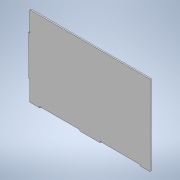
# Autodesk Inventor part: Base lateral
Saved by Autodesk Inventor 2020 (Build 240168000, 168)
## iProperties
Created: 2020-03-15
Part Number: Base lateral
Material: Genérico
Document SubType Name: Modeling
Designer: JRoCC97
Density: 1 g/cm^3
Appearance: Valor por defecto
Author: JRoCC97
Autodesk Inventor part; units mm, degrees
ref_plane "YZ Plane" through (0, 0, 0) normal (1, 0, 0) x (0, 1, 0)
ref_plane "XZ Plane" through (0, 0, 0) normal (0, 1, 0) x (-1, 0, 0)
ref_plane "XY Plane" through (0, 0, 0) normal (0, 0, 1) x (1, 0, 0)
sketch "Boceto1" plane through (0, 0, 0) normal (0, 0, 1) x (1, 0, 0)
  line L0 (0, 200) -> (300, 200)
  line L1 (300, 200) -> (300, 0)
  line L2 (25, 0) -> (25, 3)
  line L3 (25, 3) -> (125, 3)
  line L4 (125, 3) -> (125, 0)
  line L5 (175, 0) -> (175, 3)
  line L6 (175, 3) -> (275, 3)
  line L7 (275, 3) -> (275, 0)
  line L8 (25, 0) -> (0, 0)
  line L9 (300, 0) -> (275, 0)
  line L10 (175, 0) -> (125, 0)
  line L11 (0, 150) -> (-3, 150)
  line L12 (-3, 150) -> (-3, 50)
  line L13 (-3, 50) -> (0, 50)
  line L14 (0, 0) -> (0, 50)
  line L15 (0, 150) -> (0, 200)
  dimension "d4" = 100
  dimension "d6" = 100
  dimension "d10" = 50
  dimension "d13" = 3
  dimension "d14" = 200
  dimension "d15" = 3
  dimension "d16" = 100
  dimension "d17" = 50
  dimension "d18" = 300
  constraints: 32 end point, 12 perpendicular, 5 parallel, 4 collinear, 2 horizontal, 2 vertical, 1 coincident
  measures "d4" distance of L2.end L3.end
  measures "d6" distance of L5.end L6.end
  measures "d10" distance between parallel lines of L5 L4
  measures "d13" distance between parallel lines of L8 L3
  measures "d14" distance between parallel lines of L0 L9
  measures "d15" distance of L11.start L11.end
  measures "d16" distance of L11.end L12.end
  measures "d17" distance between parallel lines of L0 L11
  measures "d18" distance between parallel lines of L15 L1
extrude "Extrusión1" add sketch "Boceto1" along normal blind 3
